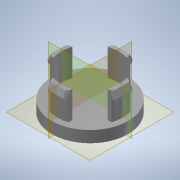
# Autodesk Inventor part: Houder kogel
Saved by Autodesk Inventor 2021 (Build 250183000, 183)
## iProperties
Manager: PJ / DCS
Company: Emmaüs Bovenbouw Aalter
Created: 2021-02-07
Part Number: Houder kogel
Material: S235
Catalog Web Link: http://emmausbovenbouw.op-weg.be/
Vendor: Emmaüsinstituut Bovenbouw Aalter
Document SubType Name: Modeling
Designer: Antho
Engineer: Declercq St.
Manufacturer: Standard
Standards Organization: Custom
Density: 7.86 g/cm^3
Appearance: Steel
Title: Algemene titel
Subject: Specifieke titel
Author: Antho
Keywords: Ruwe Ø xxxxx
Comments: Opmerking
Autodesk Inventor part; units mm, degrees
sketch "Sketch1" plane through (0, 0, 0) normal (0, 0, 1) x (1, 0, 0)
  line L0 (0, 2.8582) -> (0, -2.8582) construction
  line L1 (-5.7775, 0) -> (5.7775, 0) construction
  circle A0 centre (0, 0) radius 10
  circle A1 centre (0, 0) radius 7.5
  dimension "d0" = 20
  dimension "d1" = 15
  constraints: 4 end point, 3 coincident, 2 centre point, 2 midpoint, 1 horizontal, 1 vertical
  measures "d0" diameter of A0
  measures "d1" diameter of A1
extrude "Extrusion1" add sketch "Sketch1" along normal blind 3 contours A0 | A1
sketch "Sketch3" plane through (0, 0, 3) normal (0, 0, 1) x (1, 0, 0)
  circle A0 centre (0, 0) radius 7.5
  circle A1 centre (0, 0) radius 8.5
  dimension "d4" = 15
  dimension "d5" = 17
  constraints: 2 centre point, 2 coincident
  measures "d4" diameter of A0
  measures "d5" diameter of A1
extrude "Extrusion2" add sketch "Sketch3" along normal blind 5.1
sketch "Sketch4" plane through (0, 0, 8.1) normal (0, 0, 1) x (1, 0, 0)
  circle A0 centre (0, 0) radius 7.5
  circle A1 centre (0, 0) radius 8.5
  circle A2 centre (0, 0) radius 7.5 projected
  line L0 (0, -7.5) -> (-2.465, -7.0833)
  line L1 (-2.465, -7.0833) -> (-2.6338, -8.0817)
  line L2 (0, -7.5) -> (2.465, -7.0833)
  line L3 (2.465, -7.0833) -> (2.6338, -8.0817)
  circle A3 centre (0, 0) radius 8.5 projected
  line L4 (2.465, -7.0833) -> (2.465, -9.0833)
  line L5 (-2.465, -7.0833) -> (-2.465, -9.0833)
  line L6 (-2.465, -7.0833) -> (-0.465, -7.0833) construction
  line L7 (-2.465, -9.0833) -> (2.465, -9.0833)
  line L8 (0, 7.5) -> (-2.465, 7.0833)
  line L9 (-2.465, 7.0833) -> (-2.465, 9.0833)
  line L10 (0, 7.5) -> (2.465, 7.0833)
  line L11 (2.465, 7.0833) -> (2.465, 9.0833)
  line L12 (2.465, 9.0833) -> (-2.465, 9.0833)
  line L13 (-7.5, 0) -> (-7.0833, -2.465)
  line L14 (-7.5, 0) -> (-7.0833, 2.465)
  line L15 (-7.0833, -2.465) -> (-9.0833, -2.465)
  line L16 (-7.0833, -2.465) -> (-5.0833, -2.465) construction
  line L17 (-7.0833, 2.465) -> (-9.0833, 2.465)
  line L18 (-7.0833, 2.465) -> (-5.0833, 2.465) construction
  line L19 (-9.0833, 2.465) -> (-9.0833, -2.465)
  line L20 (7.5, 0) -> (7.0833, 2.465)
  line L21 (7.5, 0) -> (7.0833, -2.465)
  line L22 (7.0833, 2.465) -> (9.0833, 2.465)
  line L23 (7.0833, -2.465) -> (9.0833, -2.465)
  line L24 (9.0833, -2.465) -> (9.0833, 2.465)
  point P0 (2.465, 7.0833)
  point P1 (-2.465, 7.0833)
  point P2 (-7.0833, -2.465)
  point P3 (-7.0833, 2.465)
  point P4 (-8.1347, -2.465)
  point P5 (-2.465, -7.0833)
  point P6 (-8.1347, 2.465)
  point P7 (-2.465, 8.1347)
  point P8 (8.1347, 2.465)
  point P9 (2.465, 8.1347)
  point P10 (8.1347, -2.465)
  point P11 (2.6338, -8.0817)
  point P12 (-2.465, -8.1347)
  point P13 (2.465, -8.1347)
  dimension "d8" = 15
  dimension "d9" = 17
  dimension "d10" = 2.5
  dimension "d11" = 2.5
  dimension "d12" = 90
  dimension "d13" = 2
  dimension "d14" = 2
  dimension "d15" = 90
  dimension "d16" = 2.5
  dimension "d17" = 2
  dimension "d18" = 2.5
  dimension "d19" = 2
  dimension "d20" = 2.5
  dimension "d21" = 2.5
  dimension "d22" = 2
  dimension "d23" = 180
  dimension "d24" = 2
  dimension "d25" = 180
  dimension "d26" = 2.5
  dimension "d27" = 2.5
  dimension "d28" = 2
  constraints: 50 end point, 7 horizontal, 5 perpendicular, 4 vertical, 3 equal length, 2 coincident, 1 point on circle, 18 other
  measures "d10" distance of L0.start L0.end
  measures "d11" distance of L0.start L2.end
  measures "d12" angle of L2 L3
  measures "d13" distance of L2.end L4.end
  measures "d14" distance of L0.end L5.end
  measures "d15" angle of L5 L6
  measures "d16" distance of L8.start L8.end
  measures "d17" distance of L8.end L9.end
  measures "d18" distance of L8.start L10.end
  measures "d19" distance of L10.end L11.end
  measures "d20" distance of L13.start L13.end
  measures "d21" distance of L13.start L14.end
  measures "d22" distance of L13.end L15.end
  measures "d23" angle of L15 L16
  measures "d24" distance of L14.end L17.end
  measures "d25" angle of L17 L18
  measures "d26" distance of L20.start L20.end
  measures "d27" distance of L20.start L21.end
  measures "d28" distance of L20.end L22.end
extrude "Extrusion3" add sketch "Sketch4" along normal blind 2 contours A0 L22 A1 L23 | A0 L9 A1 L11 | L22 L24 L23 A1 | L4 A1 L5 A0 | A1 L9 L12 L11 | L4 L7 L5 A1 | A0 L15 A1 L17 | A1 L15 L19 L17
extrude "Extrusion4" cut sketch "Sketch4" against normal blind 5.1 contours A0 L11 A1 L22 | L23 A1 L3 A0 | L3 A1 L4 | A0 L17 A1 L9 | L1 A1 L15 A0 | L5 A1 L1
chamfer "Chamfer1" distance 0.75 distance2 1.5 1 edges at (0, -9.0833, 10.1) measured on face at (0, -8.5833, 10.1)
chamfer "Chamfer2" distance 0.75 distance2 1.5 1 edges at (9.0833, 0, 10.1) measured on face at (8.5833, 0, 10.1)
chamfer "Chamfer3" distance 0.75 distance2 1.5 1 edges at (0, 9.0833, 10.1) measured on face at (0, 8.5833, 10.1)
chamfer "Chamfer4" distance 0.75 distance2 1.5 1 edges at (-9.0833, 0, 10.1) measured on face at (-8.5833, 0, 10.1)
chamfer "Chamfer5" distance 0.5 angle 45 8 edges at (2.465, -8.7083, 9.35) (-2.465, -8.7083, 9.35) (-8.7083, -2.465, 9.35) (-8.7083, 2.465, 9.35) (-2.465, 8.7083, 9.35) (2.465, 8.7083, 9.35) (8.7083, -2.465, 9.35) (8.7083, 2.465, 9.35)
chamfer "Chamfer6" distance 0.3 angle 45 3 edges at (9.0833, 0, 8.1) (8.9288, -2.3268, 8.1) (8.9288, 2.3268, 8.1)
chamfer "Chamfer7" distance 0.3 angle 45 3 edges at (0, -9.0833, 8.1) (-2.3268, -8.9288, 8.1) (2.3268, -8.9288, 8.1)
chamfer "Chamfer8" distance 0.3 angle 45 3 edges at (-8.9288, -2.3268, 8.1) (-8.9288, 2.3268, 8.1) (-9.0833, 0, 8.1)
chamfer "Chamfer9" distance 0.3 angle 45 3 edges at (-2.3268, 8.9288, 8.1) (2.3268, 8.9288, 8.1) (0, 9.0833, 8.1)
body "Solid1"
